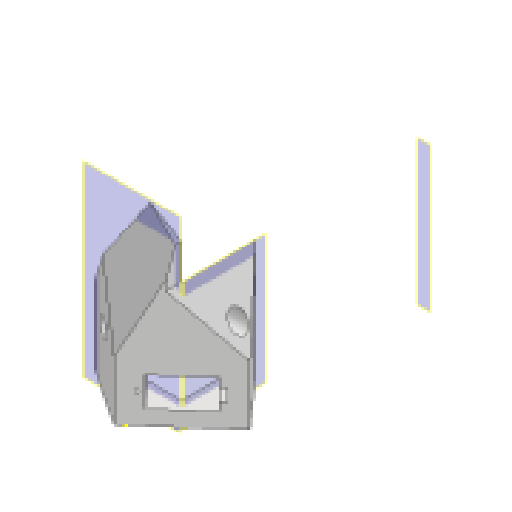
# Autodesk Inventor part: Thumb Base2
Saved by Autodesk Inventor 2025 (Build 290162010, 162A)
## iProperties
Created: 2024-12-05
Part Number: Thumb Base2
Material: Generic
Document SubType Name: Modeling
Designer: ALEXANDERNICHOLS
Density: 1 g/cm^3
Appearance: Default
Mass: 15.3387 g
Surface Area: 59.6231 cm^2
Volume: 15.3387 cm^3
Author: ALEXANDERNICHOLS
Autodesk Inventor part; units mm, degrees
ref_plane "YZ Plane" through (0, 0, 0) normal (1, 0, 0) x (0, 1, 0)
ref_plane "XZ Plane" through (0, 0, 0) normal (0, 1, 0) x (-1, 0, 0)
ref_plane "XY Plane" through (0, 0, 0) normal (0, 0, 1) x (1, 0, 0)
sketch "Sketch1" plane through (0, 0, 0) normal (0, 1, 0) x (-1, 0, 0)
  line L0 (0, 0) -> (38.1, -25.4)
  line L1 (38.1, -25.4) -> (0, -25.4)
  line L2 (0, -25.4) -> (0, -57.5469)
  line L3 (0, -57.5469) -> (-28.575, -25.4)
  line L4 (-28.575, -25.4) -> (0, 0)
  dimension "d0" = 38.1
  dimension "d2" = 25.4
  dimension "d3" = 28.575
  constraints: 10 end point, 1 horizontal, 1 horizontal alignment, 1 perpendicular, 1 vertical, 1 vertical alignment
  measures "d0" horizontal distance of L0.start L0.end
  measures "d2" distance from line of L1 L0.start
  measures "d3" horizontal distance of L3.end L0.start
extrude "Extrusion1" add sketch "Sketch1" along normal blind 25.4
sketch "Sketch2" plane through (0, 25.4, 0) normal (0, 1, 0) x (1, 0, 0)
  line L0 (-38.1, 25.4) -> (0, 0) projected
  line L1 (-11.9592, 7.9728) -> (19.3376, 35.7921)
  line L2 (0, 0) -> (28.575, 25.4) projected
  line L3 (28.575, 25.4) -> (0, 57.5469) projected
  point P0 (0, 25.4)
  dimension "d6" = 5.08
  constraints: 2 end point, 2 point on line, 1 parallel
  measures "d6" distance from line of L1 point (0, 25.4)
extrude "Extrusion2" cut sketch "Sketch2" against normal blind 49.2125
sketch "Sketch3" plane through (19.3376, 0, -35.7921) normal (0.6643638, 0, 0.7474093) x (0.7474093, 0, -0.6643638)
  line L0 (-32.3668, 19.05) -> (-9.5068, 19.05)
  line L1 (-9.5068, 19.05) -> (-9.5068, 6.35)
  line L2 (-9.5068, 6.35) -> (-32.3668, 6.35)
  line L3 (-32.3668, 6.35) -> (-32.3668, 19.05)
  line L4 (0, 25.4) -> (0, 0) projected
  line L5 (-41.8736, 25.4) -> (0, 25.4) projected
  point P0 (-38.2321, 0)
  point P1 (-9.5068, 12.7)
  point P2 (0, 12.7)
  point P3 (-20.9368, 19.05)
  point P4 (-20.9368, 25.4)
  dimension "d9" = 12.7
  dimension "d10" = 22.86
  constraints: 8 end point, 4 midpoint, 2 parallel, 1 horizontal, 1 horizontal alignment, 1 perpendicular, 1 vertical alignment
  measures "d9" distance between parallel lines of L0 L2
  measures "d10" distance of L0.start L0.end
extrude "Extrusion3" cut sketch "Sketch3" against normal blind 82.55
sketch "Sketch4" plane through (19.3376, 0, -35.7921) normal (0.6643638, 0, 0.7474093) x (0.7474093, 0, -0.6643638)
  point P0 (-38.2321, 0)
sketch "Sketch5" plane through (19.3376, 0, -35.7921) normal (0.6643638, 0, 0.7474093) x (0.7474093, 0, -0.6643638)
  line L0 (-9.5068, 6.35) -> (-9.5068, 19.05) projected
  line L1 (-9.5068, 15.24) -> (-6.9668, 15.24)
  line L2 (-6.9668, 15.24) -> (-6.9668, 10.16)
  line L3 (-6.9668, 10.16) -> (-9.5068, 10.16)
  line L4 (-9.5068, 10.16) -> (-9.5068, 15.24)
  point P0 (-38.2321, 0)
  point P1 (-6.9668, 12.7)
  point P2 (-9.5068, 12.7)
  dimension "d13" = 2.54
  dimension "d14" = 5.08
  constraints: 8 end point, 2 midpoint, 2 parallel, 1 horizontal, 1 horizontal alignment, 1 perpendicular, 1 point on line
  measures "d13" distance of L2.end L3.end
  measures "d14" distance of L1.end L2.end
extrude "Extrusion4" cut sketch "Sketch5" against normal blind 36.5125
sketch "Sketch7" plane through (0, 0, -25.4) normal (0, 0, -1) x (-1, 0, 0)
  line L0 (0, 25.4) -> (38.1, 25.4) projected
  line L1 (38.1, 0) -> (38.1, 31.4433) projected
  line L2 (38.1, 31.4433) -> (13.5942, 73.8886) projected
  line L3 (0, 66.04) -> (0, 19.05) projected
  line L4 (13.5942, 73.8886) -> (0, 66.04) projected
  point P0 (0, 0)
extrude "Extrusion6" add sketch "Sketch7" against normal blind 20.6375
sketch "Sketch8" plane through (-38.1, 25.4, -4.7625) normal (0, -1, 0) x (1, 0, 0)
  line L0 (0, -20.6375) -> (26.1408, -3.2103) projected
  line L1 (26.1408, -3.2103) -> (38.1, -13.8407) projected
  line L2 (38.1, -13.8407) -> (38.1, 0) projected
  line L3 (0, 0) -> (38.1, 0) projected
  line L4 (0, -20.6375) -> (0, 0) projected
  point P0 (38.1, 4.7625)
extrude "Extrusion7" cut sketch "Sketch8" against normal blind 74.6125
sketch "Sketch9" plane through (0, 25.4, -25.4) normal (1, 0, 0) x (0, 0, -1)
  line L0 (0, 0) -> (-6.7968, 0) projected
  line L1 (-17.4272, -25.4) -> (-17.4272, 47.5446) projected
  line L2 (0, 0) -> (-17.4272, 0)
  line L3 (-17.4272, 0) -> (0, 48.4886)
  line L4 (0, 48.4886) -> (-17.4272, 48.4886)
  line L5 (-17.4272, 48.4886) -> (-17.4272, 0)
  point P0 (-25.4, -25.4)
  constraints: 8 end point, 1 collinear, 1 parallel, 1 perpendicular, 1 point on line, 1 other
extrude "Extrusion8" cut sketch "Sketch9" against normal blind 92.075
sketch "Sketch10" plane through (0, 25.4, 0) normal (0, 1, 0) x (1, 0, 0)
  line L0 (0, 25.4) -> (0, 18.6032) projected
  line L1 (0, 18.6032) -> (19.3376, 35.7921) projected
  line L2 (19.3376, 35.7921) -> (0, 57.5469) projected
  line L3 (0, 57.5469) -> (0, 25.4) projected
  line L4 (5.08, 51.054) -> (5.08, 24.93) projected
  line L5 (5.08, 24.93) -> (5.08, 23.1187) projected
  line L6 (5.08, 52.3795) -> (5.08, 51.054) projected
  point P0 (0, 0)
extrude "Extrusion9" add sketch "Sketch10" along normal blind 25.4
ref_plane "Work Plane1" through (0, -6.35, -128.016) normal (0, 0, -1) x (0, 1, 0)
sketch "Sketch11" plane through (0, -6.35, -128.016) normal (0, 0, -1) x (0, 1, 0)
  line L0 (57.15, 19.3376) -> (57.15, 0) projected
  line L1 (57.15, 0) -> (31.75, 19.3376)
  line L2 (57.15, 19.3376) -> (6.35, 19.3376) projected
  line L3 (31.75, 19.3376) -> (57.15, 19.3376)
  line L4 (57.15, 19.3376) -> (57.15, 0)
  point P0 (6.35, 0)
  dimension "d27" = 25.4
  constraints: 6 end point, 1 horizontal, 1 midpoint, 1 perpendicular
  measures "d27" distance from line of L0 L1.end
extrude "Extrusion10" cut sketch "Sketch11" against normal blind 209.55
sketch "Sketch12" plane through (0, 0, -57.5469) normal (-1, 0, 0) x (0, 0, 1)
  circle A0 centre (19.3199, 35.56) radius 1.778
  line L0 (6.4929, 66.04) -> (6.4929, 0) projected
  line L1 (0, 50.8) -> (32.1469, 50.8) projected
  point P0 (57.5469, 0)
  dimension "d30" = 3.556
  dimension "d31" = 12.827
  dimension "d32" = 15.24
  constraints: 1 centre point
  measures "d30" diameter of A0
  measures "d31" distance from line of A0.centre L0
  measures "d32" distance from line of L1 A0.centre
extrude "Extrusion11" cut sketch "Sketch12" against normal blind 209.55
ref_plane "Work Plane2" through (2.54, 0, -57.5469) normal (-1, 0, 0) x (0, 0, 1)
sketch "Sketch13" plane through (2.54, 0, -57.5469) normal (-1, 0, 0) x (0, 0, 1)
  circle A0 centre (19.3199, 35.56) radius 1.778 projected
  circle A1 centre (19.3199, 35.56) radius 3.81
  point P0 (57.5469, 0)
  dimension "d36" = 7.62
  constraints: 1 centre point, 1 coincident
  measures "d36" diameter of A1
extrude "Extrusion12" cut sketch "Sketch13" against normal blind 209.55 contours A0 | A1
sketch "Sketch14" plane through (0, 0, -25.4) normal (0, 0, -1) x (-1, 0, 0)
  circle A0 centre (25.4, 25.4) radius 1.778
  line L0 (38.1, 0) -> (38.1, 31.4433) projected
  line L1 (0, 0) -> (38.1, 0) projected
  dimension "d39" = 3.556
  dimension "d40" = 12.7
  dimension "d41" = 25.4
  constraints: 1 centre point
  measures "d39" diameter of A0
  measures "d40" distance from line of L0 A0.centre
  measures "d41" distance from line of L1 A0.centre
extrude "Extrusion13" cut sketch "Sketch14" against normal blind 115.8875
ref_plane "Work Plane3" through (0, 0, -22.86) normal (0, 0, -1) x (-1, 0, 0)
sketch "Sketch15" plane through (0, 0, -22.86) normal (0, 0, -1) x (-1, 0, 0)
  circle A0 centre (25.4, 25.4) radius 1.778 projected
  circle A1 centre (25.4, 25.4) radius 3.81
  point P0 (0, 0)
  dimension "d45" = 7.62
  constraints: 1 centre point, 1 coincident
  measures "d45" diameter of A1
extrude "Extrusion14" cut sketch "Sketch15" against normal blind 115.8875
sketch "Sketch16" plane through (0, 0, 0) normal (0, -1, 0) x (1, 0, 0)
  circle A0 centre (-11.9592, -15.5928) radius 1.778 projected
  point P0 (0, 0)
extrude "Extrusion15" cut sketch "Sketch16" against normal blind 15.24
sketch "Sketch17" plane through (-11.9592, 0, -7.9728) normal (0.6643638, 0, 0.7474093) x (0.7474093, 0, -0.6643638)
  circle A0 centre (6.9668, 12.8573) radius 0.889
  circle A1 centre (34.9068, 12.8573) radius 0.889
  line L0 (32.3668, 6.35) -> (9.5068, 6.35) projected
  point P0 (3.6416, 0)
  point P1 (20.9368, 6.35)
  dimension "d50" = 27.94
  dimension "d51" = 1.778
  dimension "d52" = 1.778
  dimension "d53" = 13.97
  constraints: 2 centre point, 1 horizontal alignment, 1 midpoint
  measures "d50" distance of A1.centre A0.centre
  measures "d51" diameter of A0
  measures "d52" diameter of A1
  measures "d53" horizontal distance of point (20.937, 6.35) A0.centre
extrude "Extrusion16" cut sketch "Sketch17" against normal blind 3.81 contours A0
sketch "Sketch19" plane through (0, 0, 0) normal (0, -1, 0) x (1, 0, 0)
  line L0 (-16.51, -25.4) -> (-14.7303, -25.4) projected
  line L1 (-16.51, -25.4) -> (-23.1531, -15.4354)
  line L2 (-29.21, -19.4733) -> (-21.59, -14.3933) projected
  line L3 (-11.43, -25.4) -> (-17.5429, -11.6953)
  line L4 (-11.9592, -7.9728) -> (-26.2667, -17.5112) projected
  line L5 (0, -25.4) -> (-38.1, -25.4) projected
  point P0 (0, 0)
  constraints: 4 end point, 2 point on line, 1 other
extrude "Extrusion18" cut sketch "Sketch19" against normal blind 7.62
chamfer "Chamfer1" distance 1.5875 angle 45 1 edges at (-17.5429, 3.81, -11.6953)
equation "\"d53\" = 0.5 * d50"
body "Solid1"
